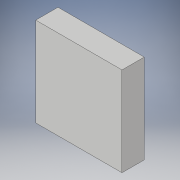
# Autodesk Inventor part: D LINK
Saved by Autodesk Inventor 2018.2 (Build 222227000, 227)
## iProperties
Created: 2018-01-27
Part Number: D LINK
Material: Generic
Document SubType Name: Modeling
Designer: matuch.michael
Density: 1 g/cm^3
Appearance: Default
Author: matuch.michael
Autodesk Inventor part; units mm, degrees
ref_plane "YZ Plane" through (0, 0, 0) normal (1, 0, 0) x (0, 1, 0)
ref_plane "XZ Plane" through (0, 0, 0) normal (0, 1, 0) x (-1, 0, 0)
ref_plane "XY Plane" through (0, 0, 0) normal (0, 0, 1) x (1, 0, 0)
sketch "Sketch1" plane through (0, 0, 0) normal (0, 0, 1) x (1, 0, 0)
  line L0 (-74.6689, 34.3341) -> (23.7561, 34.3341)
  line L1 (23.7561, 34.3341) -> (23.7561, -67.2659)
  line L2 (23.7561, -67.2659) -> (-74.6689, -67.2659)
  line L3 (-74.6689, -67.2659) -> (-74.6689, 34.3341)
  point P0 (0, 0)
  dimension "d0" = 98.425
  dimension "d1" = 101.6
  constraints: 8 end point, 2 parallel, 1 horizontal, 1 perpendicular
  measures "d0" distance of L0.start L0.end
  measures "d1" distance of L0.end L1.end
extrude "Extrusion1" add sketch "Sketch1" along normal blind 25.4
body "Solid1"
